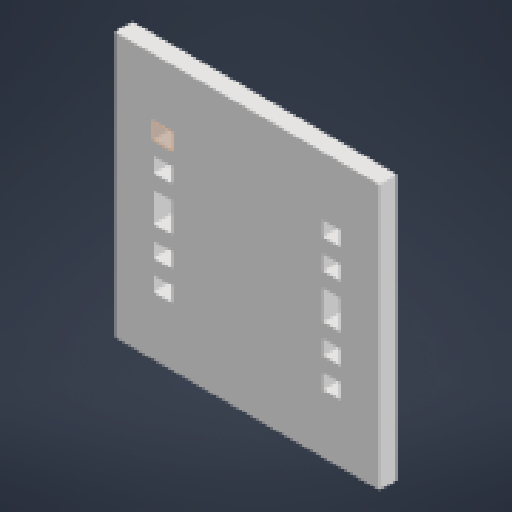
# Autodesk Inventor part: ScrewPlateLarge
Saved by Autodesk Inventor 2027 (Build 310192000, 192)
## iProperties
Created: 2026-04-15
Part Number: ScrewPlateLarge
Material: Generic
Document SubType Name: Modeling
Designer: Tueha
Density: 1 g/cm^3
Appearance: Default
Author: Tueha
Autodesk Inventor part; units mm, degrees
ref_plane "YZ Plane" through (0, 0, 0) normal (1, 0, 0) x (0, 1, 0)
ref_plane "XZ Plane" through (0, 0, 0) normal (0, 1, 0) x (-1, 0, 0)
ref_plane "XY Plane" through (0, 0, 0) normal (0, 0, 1) x (1, 0, 0)
ref_plane "Work Plane1" through (-28.4751, 43.9677, 58.8284) normal (0, 0, 1) x (1, 0, 0)
sketch "Sketch1" plane through (-28.4751, 43.9677, 58.8284) normal (0, 0, 1) x (1, 0, 0)
  line L0 (-16.2, 22.5) -> (73.8, 22.5)
  line L1 (73.8, 22.5) -> (73.8, -67.5)
  line L2 (73.8, -67.5) -> (-16.2, -67.5)
  line L3 (-16.2, -67.5) -> (-16.2, 22.5)
  line L4 (-3, -2.5) -> (3, -2.5) projected
  line L5 (3, -2.5) -> (3, 2.5) projected
  line L6 (3, 2.5) -> (-3, 2.5) projected
  line L7 (-3, 2.5) -> (-3, -2.5) projected
  line L8 (-3, -12.5) -> (3, -12.5) projected
  line L9 (3, -12.5) -> (3, -7.5) projected
  line L10 (3, -7.5) -> (-3, -7.5) projected
  line L11 (-3, -7.5) -> (-3, -12.5) projected
  line L12 (-3, -27.5) -> (3, -27.5) projected
  line L13 (3, -27.5) -> (3, -17.5) projected
  line L14 (3, -17.5) -> (-3, -17.5) projected
  line L15 (-3, -17.5) -> (-3, -27.5) projected
  line L16 (-3, -37.5) -> (3, -37.5) projected
  line L17 (3, -37.5) -> (3, -32.5) projected
  line L18 (3, -32.5) -> (-3, -32.5) projected
  line L19 (-3, -32.5) -> (-3, -37.5) projected
  line L20 (-3, -47.5) -> (3, -47.5) projected
  line L21 (3, -47.5) -> (3, -42.5) projected
  line L22 (3, -42.5) -> (-3, -42.5) projected
  line L23 (-3, -42.5) -> (-3, -47.5) projected
  line L24 (54.6, -47.5) -> (60.6, -47.5) projected
  line L25 (60.6, -47.5) -> (60.6, -42.5) projected
  line L26 (60.6, -42.5) -> (54.6, -42.5) projected
  line L27 (54.6, -42.5) -> (54.6, -47.5) projected
  line L28 (54.6, -32.5) -> (54.6, -37.5) projected
  line L29 (54.6, -37.5) -> (60.6, -37.5) projected
  line L30 (60.6, -37.5) -> (60.6, -32.5) projected
  line L31 (60.6, -32.5) -> (54.6, -32.5) projected
  line L32 (54.6, -32.5) -> (54.6, -37.5) projected
  line L33 (54.6, -27.5) -> (60.6, -27.5) projected
  line L34 (60.6, -27.5) -> (60.6, -17.5) projected
  line L35 (60.6, -17.5) -> (54.6, -17.5) projected
  line L36 (54.6, -17.5) -> (54.6, -27.5) projected
  line L37 (54.6, -12.5) -> (60.6, -12.5) projected
  line L38 (60.6, -12.5) -> (60.6, -7.5) projected
  line L39 (60.6, -7.5) -> (54.6, -7.5) projected
  line L40 (54.6, -7.5) -> (54.6, -12.5) projected
  line L41 (54.6, -2.5) -> (60.6, -2.5) projected
  line L42 (60.6, -2.5) -> (60.6, 2.5) projected
  line L43 (60.6, 2.5) -> (54.6, 2.5) projected
  line L44 (54.6, 2.5) -> (54.6, -2.5) projected
  point P0 (28.4751, -43.9677)
  point P1 (0, 2.5)
  point P2 (-3, 0)
  dimension "d0" = 90
  dimension "d1" = 90
  dimension "d2" = 20
  dimension "d3" = 13.2
  constraints: 8 end point, 2 midpoint, 2 parallel, 1 horizontal, 1 perpendicular
  measures "d0" distance of L1.end L2.end
  measures "d1" distance of L0.end L1.end
  measures "d2" distance from line of L0 point (0, 2.5)
  measures "d3" distance from line of L3 point (-3, 0)
extrude "Extrusion1" add sketch "Sketch1" against normal blind 6
body "Solid1"
